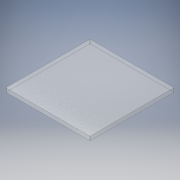
# Autodesk Inventor part: BT403_trajan20_21
Saved by Autodesk Inventor 2022.2 (Build 262287000, 287)
## iProperties
Company: HTBLA Kaindorf
RuleStatus: InUse
Created: 2022-08-21
Part Number: BT403_trajan20_21
Project: Zeichenmaschine_v2
Material: Acryl
Description: papierplatte_plexi
Document SubType Name: Modeling
Designer: trajan20
Density: 1.188 g/cm^3
Appearance: Transparent - farblos
Mass: 523.898 g
Surface Area: 965.811 cm^2
Volume: 440.991 cm^3
AfterDocNew0: iProperties-Editor_aufrufen
Author: jan
Keywords: 2021
Autodesk Inventor part; units mm, degrees
ref_plane "YZ Plane" through (0, 0, 0) normal (1, 0, 0) x (0, 1, 0)
ref_plane "XZ Plane" through (0, 0, 0) normal (0, 1, 0) x (-1, 0, 0)
ref_plane "XY Plane" through (0, 0, 0) normal (0, 0, 1) x (1, 0, 0)
sketch "Skizze3" plane through (0, 0, 0) normal (0, 0, 1) x (1, 0, 0)
  line L0 (0, 0) -> (-210, 0)
  line L1 (-210, 0) -> (-210, 210)
  line L2 (-210, 210) -> (0, 210)
  line L3 (0, 210) -> (0, 0)
  dimension "d4" = 210
  dimension "d5" = 210
  constraints: 8 end point, 2 parallel, 1 horizontal, 1 perpendicular
  measures "d4" distance between parallel lines of L2 L0
  measures "d5" distance between parallel lines of L1 L3
extrude "Extrusion3" add sketch "Skizze3" along normal blind 10
fillet "Rundung1" radius 1 4 edges at (-210, 210, 5) (-210, 0, 5) (0, 0, 5) (0, 210, 5)
equation "\"d5\" = d4"
